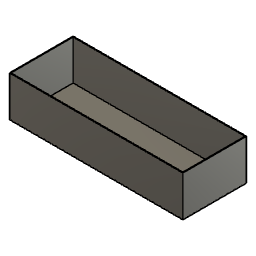
LaerCover v2 (Autodesk Fusion 360 design; units mm, degrees)
Autodesk Fusion 360 part; units mm, degrees
sketch "Skizze1" plane through (0, 0, 0) normal (0, 1, 0) x (1, 0, 0)
  line L0 (108, 39) -> (-108, 39)
  line L1 (-108, 39) -> (-108, -39)
  line L2 (-108, -39) -> (108, -39)
  line L3 (108, -39) -> (108, 39)
  line L4 (108, 39) -> (-108, -39) construction
  line L5 (-108, 39) -> (108, -39) construction
  line L6 (109, 40) -> (-109, 40)
  line L7 (-109, 40) -> (-109, -40)
  line L8 (-109, -40) -> (109, -40)
  line L9 (109, -40) -> (109, 40)
  line L10 (109, 40) -> (-109, -40) construction
  line L11 (-109, 40) -> (109, -40) construction
  dimension "d4" = 216
  dimension "d5" = 78
  dimension "d6" = 218
  dimension "d7" = 80
  constraint horizontal L0
  constraint perpendicular L0 L1
  constraint parallel L0 L2
  constraint parallel L1 L3
  constraint coincident L4 origin
  constraint coincident L5 origin
  constraint horizontal L6
  constraint perpendicular L6 L7
  constraint parallel L6 L8
  constraint parallel L7 L9
  constraint coincident L10 origin
  constraint coincident L11 origin
  measures "d4" distance of L1.end L2.end
  measures "d5" distance of L0.end L1.end
  measures "d6" distance of L7.end L8.end
  measures "d7" distance of L6.end L7.end
extrude "Extrusion1" add sketch "Skizze1" along normal blind 1 contours L0 L1 L2 L3 | L6 L7 L8 L9
extrude "Extrusion2" add sketch "Skizze1" along normal blind 51
